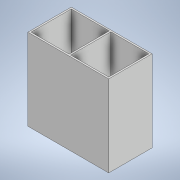
# Autodesk Inventor part: MagicBox_slim_separator
Saved by Autodesk Inventor 2020 (Build 240168000, 168)
## iProperties
Created: 2020-05-20
Part Number: MagicBox_slim_separator
Material: Generic
Document SubType Name: Modeling
Designer: user
Density: 1 g/cm^3
Appearance: Default
Author: user
## iProperties of the stored document _3DPrint.ipt
Created: 2020-05-20
Part Number: _3DPrint
Material: Generic
Document SubType Name: Modeling
Designer: user
Density: 1 g/cm^3
Appearance: Default
Author: user
Autodesk Inventor part; units mm, degrees
ref_plane "YZ Plane" through (0, 0, 0) normal (1, 0, 0) x (0, 1, 0)
ref_plane "XZ Plane" through (0, 0, 0) normal (0, 1, 0) x (-1, 0, 0)
ref_plane "XY Plane" through (0, 0, 0) normal (0, 0, 1) x (1, 0, 0)
sketch "Sketch1" plane through (0, 0, 0) normal (0, 1, 0) x (-1, 0, 0)
  line L0 (4.0152, 32.5375) -> (-70.4848, 32.5375)
  line L1 (-70.4848, 32.5375) -> (-70.4848, -7.4625)
  line L2 (-70.4848, -7.4625) -> (4.0152, -7.4625)
  line L3 (4.0152, -7.4625) -> (4.0152, 32.5375)
  point P0 (0, 0)
  dimension "d0" = 74.5
  dimension "d1" = 40
  constraints: 8 end point, 2 parallel, 1 horizontal, 1 perpendicular
  measures "d0" distance of L2.end L1.end
  measures "d1" distance of L1.end L0.end
extrude "Extrusion1" add sketch "Sketch1" along normal blind 75
sketch "Sketch3" plane through (0, 75, 0) normal (0, 1, 0) x (1, 0, 0)
  line L0 (-2.5152, 5.9625) -> (32.4848, 5.9625)
  line L1 (32.4848, 5.9625) -> (32.4848, -31.0375)
  line L2 (32.4848, -31.0375) -> (-2.5152, -31.0375)
  line L3 (-2.5152, -31.0375) -> (-2.5152, 5.9625)
  line L4 (33.9848, 5.9625) -> (68.9848, 5.9625)
  line L5 (68.9848, 5.9625) -> (68.9848, -31.0375)
  line L6 (68.9848, -31.0375) -> (33.9848, -31.0375)
  line L7 (33.9848, -31.0375) -> (33.9848, 5.9625)
  line L8 (70.4848, 7.4625) -> (-4.0152, 7.4625) projected
  line L9 (70.4848, -32.5375) -> (70.4848, 7.4625) projected
  line L10 (-4.0152, -32.5375) -> (70.4848, -32.5375) projected
  line L11 (-4.0152, 7.4625) -> (-4.0152, -32.5375) projected
  point P0 (0, 0)
  dimension "d10" = 1.5
  dimension "d11" = 1.5
  dimension "d12" = 1.5
  dimension "d13" = 1.5
  dimension "d14" = 1.5
  dimension "d15" = 35
  dimension "d16" = 35
  constraints: 16 end point, 4 parallel, 2 horizontal, 2 perpendicular, 2 point on line
  measures "d10" distance between parallel lines of L0 L8
  measures "d11" distance between parallel lines of L7 L1
  measures "d12" distance between parallel lines of L9 L5
  measures "d13" distance between parallel lines of L10 L6
  measures "d14" distance between parallel lines of L3 L11
  measures "d15" distance between parallel lines of L1 L3
  measures "d16" distance between parallel lines of L5 L7
extrude "Extrusion3" cut sketch "Sketch3" against normal blind 73.5 contours L4 L5 L6 L7
extrude "Extrusion4" cut sketch "Sketch3" against normal blind 73.5 contours L0 L1 L2 L3
equation "\"d11\" = d10"
equation "\"d12\" = d10"
equation "\"d14\" = d10"
equation "\"d15\" = d16"
body "Solid1"
